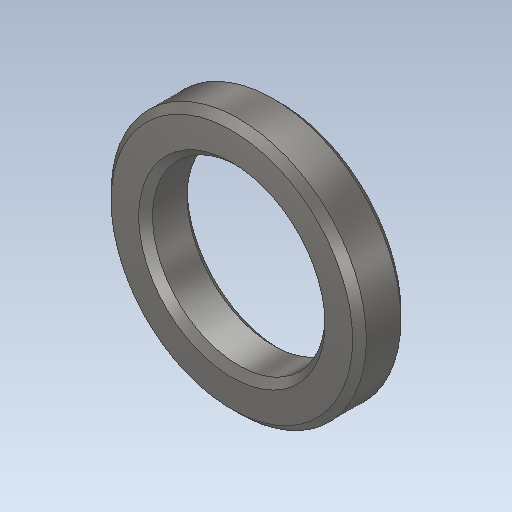
# Autodesk Inventor part: Cartesian2_BallBearing_25x37x7
Saved by Autodesk Inventor 2020 (Build 240168000, 168)
## iProperties
Created: 2020-08-24
Part Number: Cartesian2_BallBearing_25x37x7
Material: Stal, węglowa
Document SubType Name: Modeling
Designer: invin
Density: 7.85 g/cm^3
Appearance: Częściowo polerowana
Mass: 30.5803 g
Surface Area: 23.0393 cm^2
Volume: 3.89557 cm^3
Author: invin
Autodesk Inventor part; units mm, degrees
ref_plane "YZ Plane" through (0, 0, 0) normal (1, 0, 0) x (0, 1, 0)
ref_plane "XZ Plane" through (0, 0, 0) normal (0, 1, 0) x (-1, 0, 0)
ref_plane "XY Plane" through (0, 0, 0) normal (0, 0, 1) x (1, 0, 0)
sketch "Szkic1" plane through (0, 0, 0) normal (0, 0, 1) x (1, 0, 0)
  circle A0 centre (0, 0) radius 12.5
  circle A1 centre (0, 0) radius 18.5
  dimension "d0" = 25
  dimension "d1" = 37
  constraints: 2 centre point, 2 coincident
  measures "d0" diameter of A0
  measures "d1" diameter of A1
extrude "Wyciągnięcie proste1" add sketch "Szkic1" along normal blind 7
chamfer "Faza1" distance 1 angle 45 4 edges at (-18.5, 0, 7) (-12.5, 0, 7) (-12.5, 0, 0) (-18.5, 0, 0)
